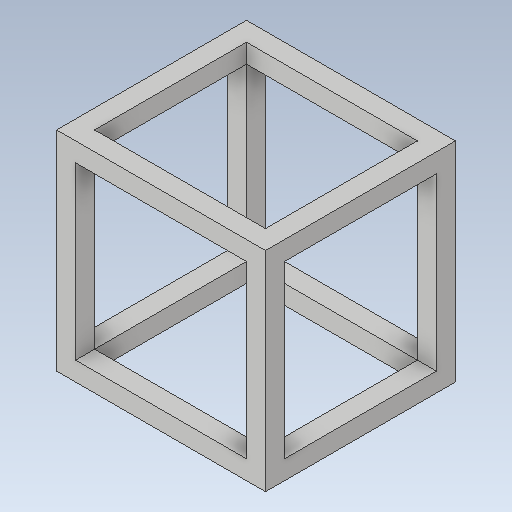
# Autodesk Inventor part: Gearbox Housing
Saved by Autodesk Inventor 2020 (Build 240168000, 168)
## iProperties
Created: 2020-10-14
Part Number: Gearbox Housing
Material: Generic
Document SubType Name: Modeling
Designer: nabee
Density: 1 g/cm^3
Appearance: Default
Author: nabee
Autodesk Inventor part; units mm, degrees
ref_plane "YZ Plane" through (0, 0, 0) normal (1, 0, 0) x (0, 1, 0)
ref_plane "XZ Plane" through (0, 0, 0) normal (0, 1, 0) x (-1, 0, 0)
ref_plane "XY Plane" through (0, 0, 0) normal (0, 0, 1) x (1, 0, 0)
sketch "Sketch1" plane through (0, 0, 0) normal (0, 0, 1) x (1, 0, 0)
  line L0 (0, 0) -> (240, 0)
  line L1 (240, 0) -> (240, 240)
  line L2 (240, 240) -> (0, 240)
  line L3 (0, 240) -> (0, 0)
  dimension "d0" = 240
  dimension "d1" = 240
  constraints: 8 end point, 2 parallel, 1 horizontal, 1 perpendicular
  measures "d0" distance of L2.end L0.start
  measures "d1" distance of L0.start L0.end
extrude "Extrusion1" add sketch "Sketch1" along normal blind 240
sketch "Sketch2" plane through (0, 0, 240) normal (0, 0, 1) x (1, 0, 0)
  line L0 (30, 210) -> (210, 210)
  line L1 (210, 210) -> (210, 30)
  line L2 (210, 30) -> (30, 30)
  line L3 (30, 30) -> (30, 210)
  line L4 (240, 240) -> (0, 240) projected
  line L5 (0, 240) -> (0, 0) projected
  line L6 (240, 0) -> (240, 240) projected
  line L7 (0, 0) -> (240, 0) projected
  dimension "d4" = 30
  dimension "d5" = 30
  dimension "d6" = 30
  dimension "d7" = 30
  constraints: 8 end point, 2 parallel, 1 horizontal, 1 perpendicular
  measures "d4" distance between parallel lines of L4 L0
  measures "d5" distance between parallel lines of L5 L3
  measures "d6" distance between parallel lines of L6 L1
  measures "d7" distance between parallel lines of L7 L2
extrude "Extrusion2" cut sketch "Sketch2" against normal blind 500 contours L0 L1 L2 L3
sketch "Sketch3" plane through (0, 240, 0) normal (0, 1, 0) x (1, 0, 0)
  line L0 (30, -30) -> (210, -30)
  line L1 (210, -30) -> (210, -210)
  line L2 (210, -210) -> (30, -210)
  line L3 (30, -210) -> (30, -30)
  line L4 (240, 0) -> (0, 0) projected
  line L5 (0, 0) -> (0, -240) projected
  line L6 (240, 0) -> (240, -240) projected
  line L7 (240, -240) -> (0, -240) projected
  dimension "d10" = 30
  dimension "d11" = 30
  dimension "d12" = 30
  dimension "d13" = 30
  constraints: 8 end point, 2 parallel, 1 horizontal, 1 perpendicular
  measures "d10" distance between parallel lines of L4 L0
  measures "d11" distance between parallel lines of L5 L3
  measures "d12" distance between parallel lines of L6 L1
  measures "d13" distance between parallel lines of L7 L2
extrude "Extrusion3" cut sketch "Sketch3" against normal blind 500 contours L0 L1 L2 L3
sketch "Sketch4" plane through (240, 0, 0) normal (1, 0, 0) x (0, 0, -1)
  line L0 (-240, 210) -> (-210, 210) projected
  line L1 (-30, 30) -> (-30, 0) projected
  line L2 (-210, 210) -> (-30, 210)
  line L3 (-30, 210) -> (-30, 30)
  line L4 (-30, 30) -> (-210, 30)
  line L5 (-210, 30) -> (-210, 210)
  point P0 (0, 0)
  constraints: 8 end point, 2 parallel, 1 horizontal, 1 perpendicular
extrude "Extrusion4" cut sketch "Sketch4" against normal blind 500
sketch "Sketch5" plane through (0, 0, 240) normal (0, 0, 1) x (1, 0, 0)
  line L0 (0, 0) -> (240, 0) projected
  line L1 (240, 240) -> (0, 240) projected
  line L2 (0, 0) -> (10, 0)
  line L3 (10, 0) -> (10, 240)
  line L4 (10, 240) -> (0, 240)
  line L5 (0, 240) -> (0, 0)
  line L6 (10, 240) -> (240, 240)
  line L7 (240, 240) -> (240, 230)
  line L8 (240, 230) -> (10, 230)
  line L9 (10, 230) -> (10, 240)
  line L10 (10, 0) -> (240, 0)
  line L11 (240, 0) -> (240, 10)
  line L12 (240, 10) -> (10, 10)
  line L13 (10, 10) -> (10, 0)
  line L14 (240, 230) -> (230, 230)
  line L15 (230, 230) -> (230, 10)
  line L16 (230, 10) -> (240, 10)
  line L17 (240, 10) -> (240, 230)
  dimension "d18" = 10
  dimension "d19" = 10
  dimension "d20" = 10
  dimension "d21" = 10
  constraints: 32 end point, 8 parallel, 4 horizontal, 4 perpendicular, 2 point on line
  measures "d18" distance of L4.end L3.end
  measures "d19" distance of L6.end L7.end
  measures "d20" distance of L10.end L11.end
  measures "d21" distance between parallel lines of L17 L15
extrude "Extrusion5" cut sketch "Sketch5" against normal blind 900 contours L5 L1 L3 L0 | L3 L12 L11 L0 | L1 L7 L8 L3 | L12 L15 L8 L17
sketch "Sketch6" plane through (10, 230, 240) normal (0, 1, 0) x (1, 0, 0)
  line L0 (0, 240) -> (220.3242, 240)
  line L1 (220.3242, 240) -> (220.3242, 230)
  line L2 (220.3242, 230) -> (0, 230)
  line L3 (0, 230) -> (0, 240)
  line L4 (0, 0) -> (220, 0) projected
  line L5 (220, 0) -> (220, 240) projected
  line L6 (0, 0) -> (220, 0)
  line L7 (220, 0) -> (220, 10)
  line L8 (220, 10) -> (0, 10)
  line L9 (0, 10) -> (0, 0)
  point P0 (-10, 240)
  dimension "d24" = 10
  dimension "d25" = 10
  constraints: 16 end point, 4 parallel, 2 horizontal, 2 perpendicular, 1 point on line
  measures "d24" distance of L0.end L1.end
  measures "d25" distance of L8.end L4.start
extrude "Extrusion6" cut sketch "Sketch6" against normal blind 900
sketch "Sketch10" plane through (10, 230, 230) normal (0, 1, 0) x (1, 0, 0)
  line L0 (0, 0) -> (0, 220) projected
  line L1 (220, 20) -> (200, 20) projected
  line L2 (0, 0) -> (220, 0)
  line L3 (220, 0) -> (220, 20)
  line L4 (220, 20) -> (0, 20)
  line L5 (0, 20) -> (0, 0)
  point P0 (-10, 230)
  constraints: 8 end point, 2 parallel, 1 horizontal, 1 perpendicular
extrude "Extrusion7" cut sketch "Sketch10" against normal blind 900
sketch "Sketch11" plane through (230, 30, 30) normal (1, 0, 0) x (0, 0, -1)
  line L0 (-180, 0) -> (0, 0) projected
  line L1 (0, 180) -> (-180, 180) projected
  line L2 (-180, 0) -> (-160, 0)
  line L3 (-160, 0) -> (-160, 180)
  line L4 (-160, 180) -> (-180, 180)
  line L5 (-180, 180) -> (-180, 0)
  point P0 (30, -30)
  dimension "d31" = 20
  constraints: 8 end point, 2 parallel, 1 horizontal, 1 perpendicular, 1 point on line
  measures "d31" distance of L4.end L3.end
extrude "Extrusion8" add sketch "Sketch11" against normal blind 220
sketch "Sketch12" plane through (30, 210, 210) normal (0, 1, 0) x (1, 0, 0)
  line L0 (180, 180) -> (180, 20) projected
  line L1 (0, 0) -> (180, 0)
  line L2 (180, 0) -> (180, 20)
  line L3 (180, 20) -> (0, 20)
  line L4 (0, 20) -> (0, 0)
  point P0 (-30, 210)
  constraints: 8 end point, 2 parallel, 1 horizontal, 1 perpendicular
extrude "Extrusion9" add sketch "Sketch12" along normal blind 20
sketch "Sketch13" plane through (30, 30, 190) normal (0, -1, 0) x (1, 0, 0)
  line L0 (0, 0) -> (-20, 0) projected
  line L1 (180, 20) -> (0, 20)
  line L2 (0, 20) -> (0, 0)
  line L3 (0, 0) -> (180, 0)
  line L4 (180, 0) -> (180, 20)
  point P0 (-30, -190)
  constraints: 8 end point, 2 parallel, 1 horizontal, 1 perpendicular
extrude "Extrusion10" add sketch "Sketch13" along normal blind 20
sketch "Sketch14" plane through (10, 230, 210) normal (0, 0, 1) x (1, 0, 0)
  line L0 (220, -20) -> (200, -20) projected
  line L1 (20, -200) -> (20, -20) projected
  line L2 (200, -20) -> (20, -20)
  line L3 (20, -20) -> (20, -200)
  line L4 (20, -200) -> (200, -200)
  line L5 (200, -200) -> (200, -20)
  point P0 (-10, -230)
  constraints: 8 end point, 2 parallel, 1 horizontal, 1 perpendicular
extrude "Extrusion11" cut sketch "Sketch14" against normal blind 20
body "Solid1"
